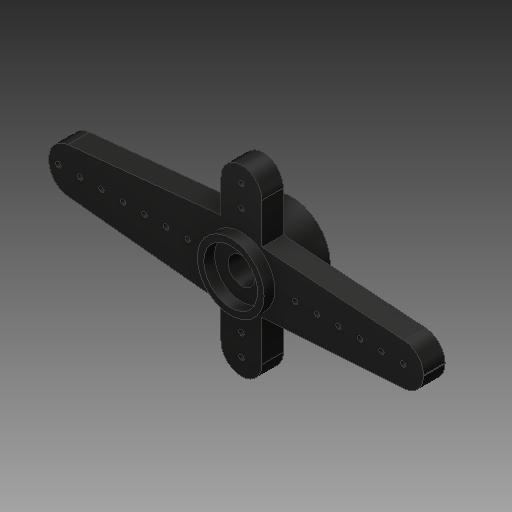
# Autodesk Inventor part: Servo_Horn_Cross_TGY
Saved by Autodesk Inventor 2019 (Build 230136000, 136)
## iProperties
Created: 2016-10-26
Part Number: Servo_Horn_Cross_TGY
Material: Generic
Document SubType Name: Modeling
Designer: Lucas
Density: 1 g/cm^3
Appearance: Glossy - Black
Mass: 0.495374 g
Surface Area: 7.96759 cm^2
Volume: 0.495374 cm^3
Author: Lucas
Autodesk Inventor part; units mm, degrees
ref_plane "YZ Plane" through (0, 0, 0) normal (1, 0, 0) x (0, 1, 0)
ref_plane "XZ Plane" through (0, 0, 0) normal (0, 1, 0) x (-1, 0, 0)
ref_plane "XY Plane" through (0, 0, 0) normal (0, 0, 1) x (1, 0, 0)
sketch "Sketch1" plane through (0, 0, 0) normal (0, 0, 1) x (1, 0, 0)
  line L0 (0, 0) -> (3.8, 0)
  line L1 (3.8, 0) -> (3.8, 17) construction
  line L2 (3.8, 17) -> (0, 17)
  line L3 (0, 17) -> (0, 0) construction
  line L4 (3.8, 17) -> (3.8, 11.325)
  line L5 (3.8, 0) -> (3.8, 5.675)
  line L6 (3.8, 8.5) -> (16.8, 8.5) construction
  line L7 (16.8, 10.45) -> (16.8, 6.55) construction
  line L8 (3.8, 5.675) -> (18.8, 6.6846)
  line L9 (3.8, 11.325) -> (18.8, 10.3154)
  line L10 (18.8, 10.3154) -> (18.8, 6.6846)
  line L11 (0, 17) -> (0, 12)
  line L12 (0, 0) -> (0, 5)
  line L13 (0, 8.5) -> (-15, 8.5) construction
  line L14 (-15, 10.5) -> (-15, 6.5) construction
  line L15 (0, 12) -> (-16, 10.4)
  line L16 (0, 5) -> (-16, 6.6)
  line L17 (-16, 10.4) -> (-16, 6.6)
  dimension "d0" = 3.8
  dimension "d1" = 17
  dimension "d2" = 5.675
  dimension "d3" = 5.675
  dimension "d4" = 13
  dimension "d5" = 3.9
  dimension "d8" = 15
  dimension "d9" = 15
  dimension "d10" = 5
  dimension "d11" = 5
  dimension "d12" = 15
  dimension "d13" = 4
  dimension "d14" = 16
  dimension "d15" = 16
  dimension "d75" = 7.701
  constraints: 36 end point, 8 point on line, 4 midpoint, 3 horizontal, 2 parallel, 2 symmetric about line, 2 vertical, 1 perpendicular
  measures "d0" distance of L2.end L1.end
  measures "d1" distance of L1.end L0.end
  measures "d2" distance of L1.end L4.end
  measures "d3" distance of L0.end L5.end
  measures "d4" distance of L6.end L6.start
  measures "d5" distance of L7.start L7.end
  measures "d8" horizontal distance of L8.end L5.end
  measures "d9" horizontal distance of L4.end L9.end
  measures "d10" distance of L2.end L11.end
  measures "d11" distance of L0.start L12.end
  measures "d12" distance of L13.start L13.end
  measures "d13" distance of L14.start L14.end
  measures "d14" horizontal distance of L11.end L15.end
  measures "d15" horizontal distance of L12.end L16.end
  measures "d75" angle of L8 L9
extrude "Horn_Body" add sketch "Sketch1" along normal blind 2
fillet "Fillet1" radius 1.9 4 edges at (3.8, 17, 1) (0, 17, 1) (0, 0, 1) (3.8, 0, 1)
fillet "Fillet2" radius 1.9 2 edges at (18.8, 6.6846, 1) (18.8, 10.3154, 1)
fillet "Fillet3" radius 2 2 edges at (-16, 10.4, 1) (-16, 6.6, 1)
sketch "Sketch2" plane through (0, 0, 0) normal (0, 0, -1) x (-1, 0, 0)
  circle A0 centre (-1.9, 8.5) radius 3.55
  line L0 (18.55, 8.5) -> (-27.4875, 8.5) construction
  line L1 (16, 8.59) -> (16, 8.41) projected
  line L2 (-1.9, 22.225) -> (-1.9, -4.7625) construction
  line L3 (-3.8, 11.325) -> (-3.8, 15.1) projected
  line L4 (0, 15.1) -> (0, 12) projected
  point P0 (0, 0)
  point P1 (16, 8.5)
  dimension "d21" = 7.1
  dimension "d22" = 3.8
  dimension "d23" = 1.9
  constraints: 4 end point, 3 point on line, 1 centre point, 1 horizontal, 1 midpoint
  measures "d21" diameter of A0
  measures "d22" distance between parallel lines of L3 L4
  measures "d23" distance between parallel lines of L4 L2
extrude "Shaft_Connector" add sketch "Sketch2" along normal blind 2.7
sketch "Sketch3" plane through (1.9, 8.5, -2.7) normal (0, 0, -1) x (-1, 0, 0)
  circle A0 centre (0, 0) radius 2.25
  point P0 (1.9, -8.5)
  dimension "d26" = 4.5
  constraints: 1 centre point
  measures "d26" diameter of A0
extrude "Shaft_Opening" cut sketch "Sketch3" against normal blind 2
sketch "Sketch4" plane through (1.9, 8.5, -0.7) normal (0, 0, -1) x (-1, 0, 0)
  circle A0 centre (0, 0) radius 1.25
  point P0 (1.9, -8.5)
  dimension "d29" = 2.5
  constraints: 1 centre point
  measures "d29" diameter of A0
extrude "Opening_Horn_FixationScrew" cut sketch "Sketch4" against normal up to surface (2.7 mm away)
sketch "Sketch6" plane through (0, 0, 2) normal (0, 0, 1) x (1, 0, 0)
  line L0 (-18.55, 8.5) -> (21.1375, 8.5) construction
  line L1 (-16, 8.59) -> (-16, 8.41) projected
  line L2 (1.9, 19.05) -> (1.9, -2.3164) construction
  line L3 (3.8, 11.325) -> (3.8, 15.1) projected
  line L4 (0, 15.1) -> (0, 12) projected
  circle A0 centre (-11.1, 8.54) radius 0.25
  circle A1 centre (-9.1, 8.5) radius 0.25
  circle A2 centre (-7.1, 8.5) radius 0.25
  circle A3 centre (-3.1, 8.5) radius 0.25
  circle A4 centre (-5.1, 8.5) radius 0.25
  circle A5 centre (-13.1, 8.5) radius 0.25
  circle A6 centre (-15.1, 8.5) radius 0.25
  circle A7 centre (6.9, 8.5) radius 0.25
  circle A8 centre (8.9, 8.5) radius 0.25
  circle A9 centre (10.9, 8.5) radius 0.25
  circle A10 centre (12.9, 8.5) radius 0.25
  circle A11 centre (14.9, 8.5) radius 0.25
  circle A12 centre (16.9, 8.5) radius 0.25
  circle A13 centre (1.9, 13.5) radius 0.25
  circle A14 centre (1.9, 15.5) radius 0.25
  circle A15 centre (1.9, 3.5) radius 0.25
  circle A16 centre (1.9, 1.5) radius 0.25
  point P0 (0, 0)
  point P1 (-16, 8.5)
  dimension "d35" = 3.8
  dimension "d36" = 1.9
  dimension "d37" = 0.5
  dimension "d38" = 0.5
  dimension "d39" = 0.5
  dimension "d41" = 0.5
  dimension "d42" = 0.5
  dimension "d43" = 5
  dimension "d44" = 2
  dimension "d46" = 2
  dimension "d47" = 2
  dimension "d48" = 2
  dimension "d49" = 0.5
  dimension "d50" = 0.5
  dimension "d51" = 2
  dimension "d52" = 2
  dimension "d53" = 0.5
  dimension "d54" = 0.5
  dimension "d55" = 0.5
  dimension "d56" = 0.5
  dimension "d57" = 0.5
  dimension "d58" = 5
  dimension "d59" = 2
  dimension "d60" = 2
  dimension "d61" = 2
  dimension "d62" = 2
  dimension "d63" = 0.5
  dimension "d64" = 2
  dimension "d65" = 0.5
  dimension "d66" = 0.5
  dimension "d67" = 0.5
  dimension "d68" = 0.5
  dimension "d69" = 5
  dimension "d70" = 2
  dimension "d71" = 5
  dimension "d72" = 2
  constraints: 17 centre point, 4 point on line, 2 end point, 1 midpoint, 1 vertical, 16 other
  measures "d35" distance between parallel lines of L3 L4
  measures "d36" distance between parallel lines of L3 L2
  measures "d37" diameter of A0
  measures "d38" diameter of A1
  measures "d39" diameter of A2
  measures "d41" diameter of A3
  measures "d42" diameter of A4
  measures "d43" distance from line of L2 A3.centre
  measures "d44" distance of A3.centre A4.centre
  measures "d46" distance of A4.centre A2.centre
  measures "d47" distance of A2.centre A1.centre
  measures "d48" horizontal distance of A1.centre A0.centre
  measures "d49" diameter of A5
  measures "d50" diameter of A6
  measures "d51" horizontal distance of A0.centre A5.centre
  measures "d52" distance of A5.centre A6.centre
  measures "d53" diameter of A7
  measures "d54" diameter of A8
  measures "d55" diameter of A9
  measures "d56" diameter of A10
  measures "d57" diameter of A11
  measures "d58" distance from line of A7.centre L2
  measures "d59" distance of A8.centre A7.centre
  measures "d60" distance of A8.centre A9.centre
  measures "d61" distance of A10.centre A9.centre
  measures "d62" distance of A11.centre A10.centre
  measures "d63" diameter of A12
  measures "d64" distance of A12.centre A11.centre
  measures "d65" diameter of A13
  measures "d66" diameter of A14
  measures "d67" diameter of A15
  measures "d68" diameter of A16
  measures "d70" distance of A14.centre A13.centre
  measures "d72" distance of A15.centre A16.centre
extrude "Connection_Holes" cut sketch "Sketch6" against normal up to surface (2 mm away)
sketch "Sketch8" plane through (0, 0, 2) normal (0, 0, 1) x (1, 0, 0)
  circle A0 centre (1.9, 8.5) radius 1.25 projected
  circle A1 centre (1.9, 8.5) radius 2.5
  circle A2 centre (1.9, 8.5) radius 3.1
  point P0 (0, 0)
  dimension "d80" = 5
  dimension "d81" = 6.2
  constraints: 2 centre point, 2 coincident
  measures "d80" diameter of A1
  measures "d81" diameter of A2
extrude "Centering_RIng" add sketch "Sketch8" along normal blind 1 contours A2
equation "\"d14\" = d15"
equation "\"d23\" = 0.5 * d22"
equation "\"d36\" = 0.5 * d35"
body "Solid1"
